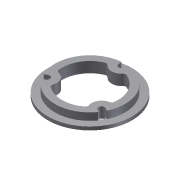
# Autodesk Inventor part: JointB0_
Saved by Autodesk Inventor 2011 SP1 (Build 150282100, 282)
## iProperties
Created: 2012-10-27
Part Number: JointB0_
Document SubType Name: Modeling
Designer: arihon
Density: 1 g/cm^3
Author: arihon
Autodesk Inventor part; units mm, degrees
ref_plane "YZ Plane" through (0, 0, 0) normal (1, 0, 0) x (0, 1, 0)
ref_plane "XZ Plane" through (0, 0, 0) normal (0, 1, 0) x (-1, 0, 0)
ref_plane "XY Plane" through (0, 0, 0) normal (0, 0, 1) x (1, 0, 0)
sketch "スケッチ1" plane through (0, 0, 0) normal (0, 0, 1) x (1, 0, 0)
  circle A0 centre (0, 0) radius 25
  dimension "d0" = 50
  constraints: 1 centre point, 1 coincident
  measures "d0" diameter of A0
extrude "押し出し1" add sketch "スケッチ1" along normal blind 5.2
sketch "スケッチ2" plane through (0, 0, 0) normal (0, 0, -1) x (-1, 0, 0)
  circle A0 centre (0, 0) radius 25 projected
  circle A1 centre (0, 0) radius 30
  dimension "d3" = 60
  constraints: 1 centre point, 1 coincident
  measures "d3" diameter of A1
extrude "押し出し2" add sketch "スケッチ2" along normal blind 2.4 contours A0 | A1
sketch "スケッチ3" plane through (0, 0, 5.2) normal (0, 0, 1) x (1, 0, 0)
  circle A0 centre (0, 0) radius 25 projected
  line L0 (0, 0) -> (0, 25)
  line L1 (0, 0) -> (21.6506, -12.5)
  line L2 (0, 0) -> (-21.6506, -12.5)
  circle A1 centre (0, 0) radius 22.5
  point P0 (0, 22.5)
  point P1 (19.4856, -11.25)
  point P2 (-19.4856, -11.25)
  dimension "d6" = 120
  dimension "d7" = 120
  dimension "d8" = 45
  constraints: 6 end point, 6 point on circle, 3 point on line, 1 centre point, 1 coincident, 1 vertical
  measures "d6" angle of L1 L0
  measures "d7" angle of L2 L1
  measures "d8" diameter of A1
hole "Hole1" at (0, 22.5, 5.2) at (19.4856, -11.25, 5.2) at (-19.4856, -11.25, 5.2) direction (0, 0, -1) diameter 4.2 end through all
shell "シェル1" thickness 5 removed faces 1 at (0, 0.0953, 5.2)
sketch "スケッチ4" plane through (0, 0, 5.2) normal (0, 0, 1) x (1, 0, 0)
  arc A0 (19.5646, -4.1504) -> (6.1879, 19.0187) centre (0, 0) ccw projected
  arc A1 (-13.3767, -14.8682) -> (13.3767, -14.8682) centre (0, 0) ccw projected
  circle A2 centre (0, 22.5) radius 2.1 projected
  circle A3 centre (0, 0) radius 25 projected
  line L0 (-2.1, 22.5) -> (2.1, 22.5)
  line L1 (2.1, 22.5) -> (2.1, 25)
  line L2 (2.1, 25) -> (-2.1, 25)
  line L3 (-2.1, 25) -> (-2.1, 22.5)
  line L4 (-18.4356, -13.0687) -> (-20.5356, -9.4313)
  line L5 (-20.5356, -9.4313) -> (-22.7006, -10.6813)
  line L6 (-22.7006, -10.6813) -> (-20.6006, -14.3187)
  line L7 (-20.6006, -14.3187) -> (-18.4356, -13.0687)
  line L8 (20.5356, -9.4313) -> (18.4356, -13.0687)
  line L9 (18.4356, -13.0687) -> (20.6006, -14.3187)
  line L10 (20.6006, -14.3187) -> (22.7006, -10.6813)
  line L11 (22.7006, -10.6813) -> (20.5356, -9.4313)
  dimension "d17" = 4.2
  dimension "d18" = 2.5
  dimension "d21" = 360
  constraints: 24 end point, 2 parallel, 1 horizontal, 1 horizontal alignment, 1 perpendicular, 32 other
  measures "d17" distance of L0.start L0.end
  measures "d18" distance of L0.end L1.end
extrude "押し出し3" cut sketch "スケッチ4" against normal up to surface (5.2 mm away) contours L0 A2 | A2 L3 A3 L1 | A3 L2 L1 | L3 L2 A3 | L5 L4 L7 A3 | A3 L6 L5 | L11 L10 A3 | A3 L9 L8 L11 | A3 L7 L6 | L10 L9 A3 picked at (0.3976, 23.0761)
sketch "スケッチ5" plane through (0, 0, 2.6) normal (0, 0, 1) x (1, 0, 0)
  arc A0 (-13.3767, -14.8682) -> (13.3767, -14.8682) centre (0, 0) ccw projected
  arc A1 (19.5646, -4.1504) -> (13.3767, -14.8682) centre (19.4856, -11.25) ccw projected
  arc A2 (19.5646, -4.1504) -> (6.1879, 19.0187) centre (0, 0) ccw projected
  arc A3 (-6.1879, 19.0187) -> (6.1879, 19.0187) centre (0, 22.5) ccw projected
  arc A4 (-6.1879, 19.0187) -> (-19.5646, -4.1504) centre (0, 0) ccw projected
  arc A5 (-13.3767, -14.8682) -> (-19.5646, -4.1504) centre (-19.4856, -11.25) ccw projected
extrude "押し出し4" cut sketch "スケッチ5" against normal through all
fillet "フィレット1" radius 2 12 edges at (-6.1879, 19.0187, 3.9) (-6.1879, 19.0187, 0.1) (6.1879, 19.0187, 3.9) (6.1879, 19.0187, 0.1) (19.5646, -4.1504, 3.9) (19.5646, -4.1504, 0.1) (13.3767, -14.8682, 3.9) (13.3767, -14.8682, 0.1) (-13.3767, -14.8682, 3.9) (-13.3767, -14.8682, 0.1) (-19.5646, -4.1504, 3.9) (-19.5646, -4.1504, 0.1)
fillet "フィレット2" radius 0.5 6 edges at (2.1, 24.9116, 2.6) (-2.1, 24.9116, 2.6) (-22.6241, -10.6372, 2.6) (-20.5241, -14.2745, 2.6) (20.5241, -14.2745, 2.6) (22.6241, -10.6372, 2.6)
